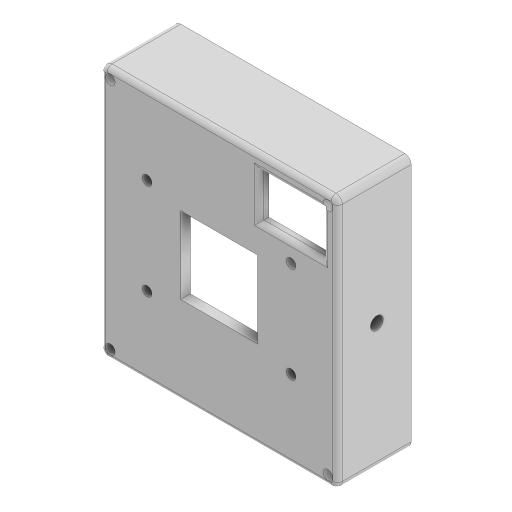
# Autodesk Inventor part: manta ray battery pack
Saved by Autodesk Inventor 2024 (Build 280153000, 153)
## iProperties
Created: 2024-01-11
Part Number: manta ray battery pack
Material: Generic
Document SubType Name: Modeling
Designer: chris
Density: 1 g/cm^3
Appearance: Default
Author: chris
Autodesk Inventor part; units mm, degrees
ref_plane "YZ Plane" through (0, 0, 0) normal (1, 0, 0) x (0, 1, 0)
ref_plane "XZ Plane" through (0, 0, 0) normal (0, 1, 0) x (-1, 0, 0)
ref_plane "XY Plane" through (0, 0, 0) normal (0, 0, 1) x (1, 0, 0)
sketch "Sketch2" plane through (0, 0, 0) normal (0, 0, 1) x (1, 0, 0)
  line L0 (0, -40) -> (0, -15)
  line L1 (0, -15) -> (-34, -15)
  line L2 (-34, -15) -> (-34, 58)
  line L3 (-34, 58) -> (34, 58)
  line L4 (34, 58) -> (34, -15)
  line L5 (34, -15) -> (0, -15)
  circle A0 centre (-34, 58) radius 1.5
  circle A1 centre (34, 58) radius 1.5
  circle A2 centre (-34, -15) radius 1.5
  circle A3 centre (34, -15) radius 1.5
  line L6 (32.5, 56.5) -> (-32.5, 56.5)
  line L7 (-32.5, 56.5) -> (-32.5, -13.5)
  line L8 (-32.5, -13.5) -> (0, -13.5)
  line L9 (0, -13.5) -> (32.5, -13.5)
  line L10 (32.5, -13.5) -> (32.5, 56.5)
  line L11 (37, -18) -> (37, 61)
  line L12 (37, 61) -> (-37, 61)
  line L13 (-37, 61) -> (-37, -18)
  line L14 (-37, -18) -> (0, -18)
  line L15 (0, -18) -> (37, -18)
  point P0 (0, 0)
  dimension "d0" = 25
  dimension "d1" = 34
  dimension "d3" = 68
  dimension "d4" = 3
  dimension "d5" = 3
  dimension "d6" = 3
  dimension "d11" = 1.5
  dimension "d13" = 3
  constraints: 32 end point, 13 perpendicular, 4 centre point, 4 coincident, 1 point on line, 1 vertical, 8 other
  measures "d0" distance of L0.start L0.end
  measures "d1" distance of L0.end L1.end
  measures "d3" distance of L2.end L3.end
  measures "d4" diameter of A0
  measures "d5" diameter of A1
  measures "d6" diameter of A2
  measures "d11" distance between parallel lines of L3 L6
  measures "d13" distance between parallel lines of L4 L11
extrude "Extrusion1" add sketch "Sketch2" along normal blind 20 contours L1 A2 L2 A0 L3 A1 L4 A3 L5 | L15 L14 L13 L12 L11
fillet "Fillet1" radius 2 4 edges at (37, -18, 10) (37, 61, 10) (-37, 61, 10) (-37, -18, 10)
sketch "Sketch3" plane through (0, 0, 20) normal (0, 0, 1) x (1, 0, 0)
  arc A0 (-37, -16) -> (-35, -18) centre (-35, -16) ccw projected
  line L0 (-35, -18) -> (35, -18) projected
  arc A1 (35, -18) -> (37, -16) centre (35, -16) ccw projected
  line L1 (37, -16) -> (37, 59) projected
  arc A2 (37, 59) -> (35, 61) centre (35, 59) ccw projected
  line L2 (35, 61) -> (-35, 61) projected
  arc A3 (-35, 61) -> (-37, 59) centre (-35, 59) ccw projected
  line L3 (-37, 59) -> (-37, -16) projected
  circle A4 centre (34, -15) radius 1.5 projected
  circle A5 centre (-34, -15) radius 1.5 projected
  circle A6 centre (-34, 58) radius 1.5 projected
  line L4 (32.5, 56.5) -> (32.5, -13.5) projected
  line L5 (32.5, -13.5) -> (-32.5, -13.5) projected
  line L6 (-32.5, -13.5) -> (-32.5, 56.5) projected
  line L7 (-32.5, 56.5) -> (32.5, 56.5) projected
  circle A7 centre (34, 58) radius 1.5 projected
  point P0 (0, 0)
extrude "Extrusion2" add sketch "Sketch3" along normal blind 3 contours L3 A3 L2 A2 L1 A1 L0 A0 | L4 L5 L6 L7
fillet "Fillet2" radius 1.5 8 edges at (36.4142, 60.4142, 23) (0, 61, 23) (-36.4142, 60.4142, 23) (-37, 21.5, 23) (-36.4142, -17.4142, 23) (0, -18, 23) (36.4142, -17.4142, 23) (37, 21.5, 23)
sketch "Sketch4" plane through (0, 0, 20) normal (0, 0, -1) x (-1, 0, 0)
  line L0 (-32.5, 56.5) -> (-32.5, -13.5) projected
  line L1 (-32.5, 56.5) -> (-12.5, 56.5)
  line L2 (32.5, 56.5) -> (-32.5, 56.5) projected
  line L3 (-12.5, 56.5) -> (-12.5, 42.5)
  line L4 (-12.5, 42.5) -> (-32.5, 42.5)
  point P0 (0, 0)
  dimension "d18" = 20
  dimension "d19" = 14
  constraints: 6 end point, 2 perpendicular, 1 point on line
  measures "d18" distance of L0.start L1.end
  measures "d19" distance of L1.end L3.end
extrude "Extrusion3" cut sketch "Sketch4" against normal blind 3
fillet "Fillet3" radius 1.5 4 edges at (12.5, 49.5, 23) (22.5, 56.5, 23) (32.5, 49.5, 23) (22.5, 42.5, 23)
sketch "Sketch6" plane through (0, 0, 23) normal (0, 0, 1) x (1, 0, 0)
  line L0 (34, -16.5) -> (-34, -16.5) projected
  line L1 (-35.5, -15) -> (-35.5, 58) projected
  line L2 (0, 21.5) -> (0, 36.5)
  line L3 (0, 36.5) -> (-15, 36.5)
  line L4 (-15, 36.5) -> (-15, 6.5)
  line L5 (-15, 6.5) -> (15, 6.5)
  line L6 (15, 6.5) -> (15, 36.5)
  line L7 (15, 36.5) -> (0, 36.5)
  line L8 (-12, 33.5) -> (0, 33.5)
  line L9 (0, 33.5) -> (12, 33.5)
  line L10 (12, 33.5) -> (12, 9.5)
  line L11 (12, 9.5) -> (-12, 9.5)
  line L12 (-12, 9.5) -> (-12, 33.5)
  line L13 (-15, 36.5) -> (-22.5, 36.5)
  circle A0 centre (-22.5, 36.5) radius 1.5
  circle A1 centre (-22.5, 6.5) radius 1.5
  circle A2 centre (22.5, 36.5) radius 1.5
  circle A3 centre (22.5, 6.5) radius 1.5
  dimension "d33" = 15
  dimension "d34" = 15
  dimension "d35" = 30
  dimension "d36" = 30
  dimension "d37" = 3
  dimension "d38" = 7.5
  dimension "d39" = 3
  dimension "d40" = 3
  constraints: 24 end point, 8 perpendicular, 4 centre point, 2 point on line, 2 symmetric about line, 1 coincident, 1 horizontal, 6 other
  measures "d33" distance of L2.start L2.end
  measures "d34" distance of L2.end L3.end
  measures "d35" distance of L3.end L4.end
  measures "d36" distance of L4.end L5.end
  measures "d37" distance between parallel lines of L3 L8
  measures "d38" distance of L3.end L13.end
  measures "d39" diameter of A0
  measures "d40" diameter of A1
extrude "Extrusion5" cut sketch "Sketch6" against normal blind 5 contours L8 L9 L10 L11 L12 | A0 | A1 | A2 | A3
sketch "Sketch7" plane through (0, 0, 0) normal (0, 0, -1) x (-1, 0, 0)
  line L0 (32.5, -13.5) -> (32.5, 56.5) projected
  line L1 (32.5, 56.5) -> (27.5, 56.5)
  line L2 (32.5, 56.5) -> (-32.5, 56.5) projected
  line L3 (27.5, 56.5) -> (29.5, 56.5)
  line L4 (29.5, 56.5) -> (29.5, 58.5)
  line L5 (29.5, 58.5) -> (25.5, 58.5)
  line L6 (25.5, 58.5) -> (25.5, 56.5)
  line L7 (29.5, 58.5) -> (31, 58.5)
  line L8 (31, 58.5) -> (31, 56.5)
  line L9 (25.5, 58.5) -> (24, 58.5)
  line L10 (24, 58.5) -> (24, 56.5)
  line L11 (0, 56.5) -> (0, 48.9008)
  line L12 (-32.5, 56.5) -> (-27.5, 56.5)
  line L13 (-32.5, 56.5) -> (32.5, 56.5)
  line L14 (-27.5, 56.5) -> (-29.5, 56.5)
  line L15 (-29.5, 56.5) -> (-29.5, 58.5)
  line L16 (-29.5, 58.5) -> (-25.5, 58.5)
  line L17 (-25.5, 58.5) -> (-25.5, 56.5)
  line L18 (-29.5, 58.5) -> (-31, 58.5)
  line L19 (-31, 58.5) -> (-31, 56.5)
  line L20 (-25.5, 58.5) -> (-24, 58.5)
  line L21 (-24, 58.5) -> (-24, 56.5)
  line L22 (24, 58.5) -> (-24, 58.5)
  point P0 (0, 0)
  dimension "d44" = 5
  dimension "d45" = 2
  dimension "d46" = 2
  dimension "d47" = 4
  dimension "d48" = 1.5
  dimension "d49" = 1.5
  constraints: 42 end point, 14 point on line, 11 symmetric about line, 4 perpendicular, 2 vertical, 1 midpoint, 1 parallel
  measures "d44" distance of L0.end L1.end
  measures "d45" distance of L1.end L3.end
  measures "d46" distance of L3.end L4.end
  measures "d47" distance of L4.end L5.end
  measures "d48" distance of L4.end L7.end
  measures "d49" distance of L5.end L9.end
extrude "Extrusion6" cut sketch "Sketch7" against normal up to surface (20 mm away)
fillet "Fillet5" radius 1.5 4 edges at (31, 58.5, 10) (31, 56.5, 10) (-31, 58.5, 10) (-31, 56.5, 10)
sketch "Sketch8" plane through (37, -16, 0) normal (1, 0, 0) x (0, 0, -1)
  line L0 (0, 77) -> (-21.5, 77) projected
  line L1 (-10.75, 77) -> (-10.75, -2)
  line L2 (-21.5, -2) -> (0, -2) projected
  circle A0 centre (-10.75, 37.5) radius 2
  point P0 (0, 16)
  dimension "d54" = 4
  constraints: 3 midpoint, 2 end point, 1 centre point
  measures "d54" diameter of A0
extrude "Extrusion7" cut sketch "Sketch8" against normal through all
body "Solid1"
